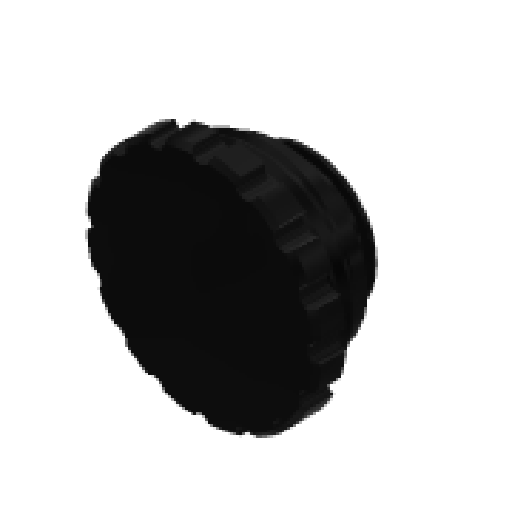
# Autodesk Inventor part: PRT - 9302 - MFLEAFPLUG - V04
Saved by Autodesk Inventor 2025.3 (Build 293356000, 356)
## iProperties
Part Number: PRT - 9302 - MFLEAFPLUG - V04
Material: Generic
Description: Leaf chamber screw plug, O-ring 12 x 1.5 on the stub, solid
Document SubType Name: Modeling
Designer: benir
Appearance: Low Gloss - Black
Author: benir
Autodesk Inventor part; units mm, degrees
ref_plane "z = boss_top + head_gap" through (0, 0, 10) normal (0, 0, 1) x (1, 0, 0)
sketch "head sketch" plane through (0, 0, 10) normal (0, 0, 1) x (1, 0, 0)
  circle A0 centre (0, 0) radius 12
  dimension "d1" = 24
  constraints: 1 centre point
  measures "d1" diameter of A0
extrude "head" add sketch "head sketch" along normal blind 3
ref_plane "z = ledge_z" through (0, 0, 4.7) normal (0, 0, 1) x (1, 0, 0)
sketch "thread body sketch" plane through (0, 0, 4.7) normal (0, 0, 1) x (1, 0, 0)
  circle A0 centre (0, 0) radius 9.75
  dimension "d5" = 19.5
  constraints: 1 centre point
  measures "d5" diameter of A0
extrude "thread body" add sketch "thread body sketch" along normal blind 5.3
ref_plane "z = chamber_h" through (0, 0, 1.5) normal (0, 0, 1) x (1, 0, 0)
sketch "stub sketch" plane through (0, 0, 1.5) normal (0, 0, 1) x (1, 0, 0)
  circle A0 centre (0, 0) radius 6.9
  dimension "d9" = 13.8
  constraints: 1 centre point
  measures "d9" diameter of A0
extrude "stub" add sketch "stub sketch" along normal blind 3.2 and the other way blind 1
sketch "thread relief sketch" plane through (0, 0, 4.7) normal (0, 0, 1) x (1, 0, 0)
  circle A0 centre (0, 0) radius 10.25
  circle A1 centre (0, 0) radius 8.8381
  dimension "d12" = 20.5
  dimension "d13" = 17.6762
  constraints: 2 centre point
  measures "d12" diameter of A0
  measures "d13" diameter of A1
extrude "thread relief" cut sketch "thread relief sketch" along normal blind 1.5
ref_plane "z = groove_z0" through (0, 0, 2.2) normal (0, 0, 1) x (1, 0, 0)
sketch "O-ring groove sketch" plane through (0, 0, 2.2) normal (0, 0, 1) x (1, 0, 0)
  circle A0 centre (0, 0) radius 7.4
  circle A1 centre (0, 0) radius 6
  dimension "d17" = 14.8
  dimension "d18" = 12
  constraints: 2 centre point
  measures "d17" diameter of A0
  measures "d18" diameter of A1
extrude "O-ring groove" cut sketch "O-ring groove sketch" along normal blind 2.1
chamfer "head chamfer" distance 0.5 angle 45 1 edges at (-12, 0, 13)
sketch "external thread groove profile" plane through (0, 0, 0) normal (0, 1, 0) x (-1, 0, 0)
  line L0 (-8.9381, 4.6827) -> (-9.85, 4.1562)
  line L1 (-9.85, 4.1562) -> (-9.85, 5.5842)
  line L2 (-9.85, 5.5842) -> (-8.9381, 5.0577)
  line L3 (-8.9381, 5.0577) -> (-8.9381, 4.6827)
  point P0 (0, 0)
  dimension "d27" = 4.6827
  dimension "d28" = 8.9381
  dimension "d29" = 4.1562
  dimension "d30" = 9.85
  dimension "d31" = 5.5842
  dimension "d32" = 9.85
  dimension "d33" = 5.0577
  dimension "d34" = 8.9381
  constraints: 8 end point
  measures "d27" vertical distance of point (0, 0) L0.start
  measures "d28" horizontal distance of point (0, 0) L0.start
  measures "d29" vertical distance of point (0, 0) L0.end
  measures "d30" horizontal distance of point (0, 0) L0.end
  measures "d31" vertical distance of point (0, 0) L1.end
  measures "d32" horizontal distance of point (0, 0) L1.end
  measures "d33" vertical distance of point (0, 0) L2.end
  measures "d34" horizontal distance of point (0, 0) L2.end
coil "M20x1.5 external thread (coil cut, RH)" sketch "external thread groove profile" operation cut axis through (0, 0, -10) along (0, 0, 1) pitch 1.5 turns 3.553186 hand right
ref_plane "z = plug_top" through (0, 0, 13) normal (0, 0, 1) x (1, 0, 0)
sketch "grip flute sketch" plane through (0, 0, 13) normal (0, 0, 1) x (1, 0, 0)
  circle A0 centre (12, 0) radius 1
  line L0 (-17, 0) -> (18, 0) projected
  point P0 (0, 0)
  dimension "d44" = 12
  dimension "d45" = 2
  constraints: 1 centre point, 1 point on line
  measures "d44" distance of point (0, 0) A0.centre
  measures "d45" diameter of A0
extrude "grip flute" cut sketch "grip flute sketch" against normal blind 3.5
pattern_circular "grip flutes" count 16 over 360 about axis through (0, 0, -10) along (0, 0, 1) of "grip flute"
sketch "Sketch9" plane through (0, 0, 13) normal (0, 0, 1) x (1, 0, 0)
  circle A0 centre (0, 0) radius 4.5
  dimension "d54" = 9
  constraints: 1 centre point, 1 coincident
  measures "d54" diameter of A0
extrude "Extrusion8" cut sketch "Sketch9" against normal through all
chamfer "stub lead-in" distance 0.3 angle 45 3 edges at (-6.9, 0, 0.5) (-4.5, 0, 0.5) (-4.5, 0, 13)
equation "\"d1\" = head_d"
equation "\"d2\" = head_h"
equation "\"d5\" = th_ext_d"
equation "\"d6\" = head_gap + boss_top - ledge_z"
equation "\"d9\" = stub_d"
equation "\"d10\" = ledge_z - chamber_h"
equation "\"d13\" = relief_d"
equation "\"d14\" = th_p"
equation "\"d18\" = groove_root_d"
equation "\"d19\" = groove_w"
equation "\"d27\" = te_zc - 0.5 * te_w_root"
equation "\"d28\" = 0.5 * th_ext_root_d"
equation "\"d29\" = te_zc - 0.5 * te_w_out"
equation "\"d30\" = te_r_out"
equation "\"d31\" = te_zc + 0.5 * te_w_out"
equation "\"d32\" = te_r_out"
equation "\"d33\" = te_zc + 0.5 * te_w_root"
equation "\"d34\" = 0.5 * th_ext_root_d"
equation "\"d35\" = th_p"
equation "\"d36\" = te_height"
equation "\"d44\" = 0.5 * head_d"
equation "\"d45\" = flute_d"
equation "\"chamber_h\" = 1.5"
equation "\"stub_len\" = 3.2"
equation "\"ledge_z\" = chamber_h + stub_len"
equation "\"th_len\" = 5"
equation "\"boss_top\" = ledge_z + th_len"
equation "\"head_gap\" = 0.3"
equation "\"head_d\" = 24"
equation "\"head_h\" = 3"
equation "\"d4\" = ledge_z"
equation "\"plug_th_clear\" = 0.25"
equation "\"th_ext_d\" = th_d - 2 * plug_th_clear"
equation "\"d8\" = chamber_h"
equation "\"well_d\" = 14.3"
equation "\"stub_clear\" = 0.25"
equation "\"stub_d\" = well_d - 2 * stub_clear"
equation "\"th_p\" = 1.5"
equation "\"th_ext_root_d\" = -2 * plug_th_clear + th_d - 1.0825 * th_p"
equation "\"groove_top_gap\" = 0.4"
equation "\"groove_w\" = 2.1"
equation "\"groove_z0\" = -groove_top_gap + ledge_z - groove_w"
equation "\"d16\" = groove_z0"
equation "\"groove_root_d\" = 12"
equation "\"th_start\" = 0.3"
equation "\"ti_w_root\" = 0.125 * th_p"
equation "\"th_clear\" = 0.15"
equation "\"th_root_d\" = th_d + 2 * th_clear"
equation "\"th_bore_d\" = -1.0825 * th_p + th_d + 2 * th_clear"
equation "\"ti_w_in\" = ti_w_root + 0.57735 * th_root_d - 1.1547 * ti_r_in"
equation "\"ti_zc\" = th_start + ledge_z + 0.5 * ti_w_in"
equation "\"te_zc\" = ti_zc - 0.5 * th_p"
equation "\"te_w_root\" = 0.25 * th_p"
equation "\"te_w_out\" = te_w_root + 1.1547 * te_r_out - 0.57735 * th_ext_root_d"
equation "\"plug_top\" = head_gap + boss_top + head_h"
equation "\"d43\" = plug_top"
equation "\"flute_d\" = 2"
equation "\"relief_d\" = 17.67625"
equation "\"te_height\" = 5.329779"
equation "\"th_d\" = 20"
equation "\"ti_r_in\" = 9.238125"
equation "\"te_r_out\" = 9.85"
body "Solid1"
